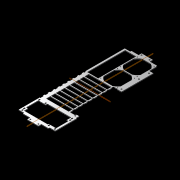
# Autodesk Inventor part: backpanel
Saved by Autodesk Inventor 2018 (Build 220112000, 112)
## iProperties
Created: 2019-10-14
Part Number: backpanel
Material: アルミニウム 6061
Document SubType Name: Modeling
Designer: gisen
Density: 2.7 g/cm^3
Appearance: アルミニウム - フラット
Author: gisen
Autodesk Inventor part; units mm, degrees
ref_plane "XY Plane" through (0, 0, 0) normal (0, 0, 1) x (1, 0, 0)
sketch "スケッチ1" plane through (0, 0, 0) normal (0, 0, 1) x (1, 0, 0)
  line L0 (-55, -225) -> (55, -225) construction
  line L1 (55, -225) -> (55, 225) construction
  line L2 (55, 225) -> (-55, 225) construction
  line L3 (-55, 225) -> (-55, -225) construction
  line L4 (-55, -225) -> (55, 225) construction
  line L5 (55, -225) -> (-55, 225) construction
  line L6 (-75, 225) -> (-55, 225)
  line L7 (-55, 225) -> (-55, 242.5)
  line L8 (-55, 242.5) -> (55, 242.5)
  line L9 (55, 242.5) -> (55, 225)
  line L10 (55, 225) -> (75, 225)
  line L11 (75, 225) -> (75, -225)
  line L12 (75, -225) -> (55, -225)
  line L13 (55, -225) -> (55, -242.5)
  line L14 (55, -242.5) -> (-55, -242.5)
  line L15 (-55, -242.5) -> (-55, -225)
  line L16 (-55, -225) -> (-75, -225)
  line L17 (-75, -225) -> (-75, 225)
  line L18 (-65, 235) -> (65, 235) construction
  line L19 (65, 235) -> (65, -235) construction
  line L20 (65, -235) -> (-65, -235) construction
  line L21 (-65, -235) -> (-65, 235) construction
  circle A0 centre (-45, 235) radius 2.25
  circle A1 centre (-65, 215) radius 2.25
  line L22 (0, 0) -> (0, 242.5) construction
  line L23 (0, 0) -> (-75, 0) construction
  circle A2 centre (45, 235) radius 2.25
  circle A3 centre (65, 215) radius 2.25
  circle A4 centre (-45, -235) radius 2.25
  circle A5 centre (-65, -215) radius 2.25
  circle A6 centre (45, -235) radius 2.25
  circle A7 centre (65, -215) radius 2.25
  dimension "d0" = 110
  dimension "d1" = 450
  dimension "d2" = 17.5
  dimension "d3" = 17.5
  dimension "d4" = 20
  dimension "d5" = 20
  dimension "d6" = 10
  dimension "d7" = 10
  dimension "d8" = 10
  dimension "d9" = 10
  dimension "d10" = 4.5
  dimension "d11" = 10
  dimension "d12" = 10
  constraints: 48 end point, 8 centre point, 6 perpendicular, 6 point on line, 6 symmetric about line, 5 parallel, 4 midpoint, 4 vertical, 3 horizontal, 1 equal radius, 6 other
  measures "d0" distance of L2.end L1.end
  measures "d1" distance of L1.end L0.end
  measures "d2" distance of L8.end L1.end
  measures "d3" distance of L0.end L13.end
  measures "d4" distance of L1.end L10.end
  measures "d5" distance of L6.start L2.end
  measures "d6" distance between parallel lines of L2 L18
  measures "d7" distance between parallel lines of L3 L21
  measures "d8" distance between parallel lines of L0 L20
  measures "d9" distance between parallel lines of L1 L19
  measures "d10" diameter of A0
  measures "d11" distance from line of L7 A0.centre
  measures "d12" distance from line of A1.centre L6
extrude "押し出し1" add sketch "スケッチ1" along normal blind 3 contours L6 L7 L8 L9 L10 L11 L12 L13 L14 L15 L16 L17 | A1 | A5 | A7
sketch "スケッチ2" plane through (0, 0, 3) normal (0, 0, 1) x (1, 0, 0)
  line L0 (-68.059, 218.004) -> (-25.879, 218.004) construction
  line L1 (-69.259, 60.324) -> (-69.259, 216.804) construction
  line L2 (-25.879, 59.124) -> (-68.059, 59.124) construction
  line L3 (-24.679, 216.804) -> (-24.679, 60.324) construction
  line L4 (-24.679, 59.124) -> (-69.259, 59.124) construction
  line L5 (-69.259, 59.124) -> (-69.259, 218.004) construction
  line L6 (-69.259, 218.004) -> (-24.679, 218.004) construction
  line L7 (-24.679, 218.004) -> (-24.679, 59.124) construction
  line L8 (-24.679, 59.124) -> (-69.259, 218.004) construction
  line L9 (-69.259, 59.124) -> (-24.679, 218.004) construction
  line L10 (-69.319, 59.064) -> (-24.619, 59.064)
  line L11 (-24.619, 59.064) -> (-24.619, 218.064)
  line L12 (-24.619, 218.064) -> (-69.319, 218.064)
  line L13 (-69.319, 218.064) -> (-69.319, 59.064)
  line L14 (-69.319, 59.064) -> (-24.619, 218.064) construction
  line L15 (-24.619, 59.064) -> (-69.319, 218.064) construction
  point P0 (0, 0)
  point P1 (-46.969, 138.564)
  point P2 (-46.969, 218.004)
  point P3 (-69.259, 138.564)
  dimension "d16" = 44.7
  dimension "d17" = 159
  constraints: 24 end point, 8 midpoint, 4 parallel, 2 horizontal, 2 perpendicular
  measures "d16" distance of L12.end L11.end
  measures "d17" distance of L11.end L10.end
extrude "押し出し2" cut sketch "スケッチ2" against normal blind 3
sketch "スケッチ3" plane through (0, 0, 3) normal (0, 0, 1) x (1, 0, 0)
  line L0 (-70.088, -102.7387) -> (-77.3126, -102.7387) construction
  line L1 (-77.3126, -92.4517) -> (-70.088, -92.4517) construction
  line L2 (-70.088, -82.3933) -> (-77.3126, -82.3933) construction
  line L3 (-77.3126, -72.1063) -> (-70.088, -72.1063) construction
  line L4 (-70.088, -61.7387) -> (-77.3126, -61.7387) construction
  line L5 (-77.3126, -51.4517) -> (-70.088, -51.4517) construction
  line L6 (-70.088, -41.3933) -> (-77.3126, -41.3933) construction
  line L7 (-77.3126, -31.1063) -> (-70.088, -31.1063) construction
  line L8 (-70.088, -20.7387) -> (-77.3126, -20.7387) construction
  line L9 (-77.3126, -10.4517) -> (-70.088, -10.4517) construction
  line L10 (-70.088, -0.3933) -> (-77.3126, -0.3933) construction
  line L11 (-77.3126, 9.8937) -> (-70.088, 9.8937) construction
  line L12 (-70.088, 20.2613) -> (-77.3126, 20.2613) construction
  line L13 (-77.3126, 30.5483) -> (-70.088, 30.5483) construction
  line L14 (-70.088, 40.6067) -> (-77.3126, 40.6067) construction
  line L15 (-77.3126, 50.8937) -> (-70.088, 50.8937) construction
  line L16 (-75, 225) -> (-75, -225) construction
  line L17 (-75, 56.064) -> (-78, 56.064)
  line L18 (-78, 56.064) -> (-78, 225)
  line L19 (-78, 225) -> (-75, 225)
  line L20 (-75, 225) -> (-75, 56.064)
  line L21 (-24.619, 59.064) -> (-69.319, 59.064) projected
  line L22 (-75, -102.7387) -> (-78, -102.7387)
  line L23 (-78, -102.7387) -> (-78, -92.4517)
  line L24 (-78, -92.4517) -> (-75, -92.4517)
  line L25 (-75, -92.4517) -> (-75, -102.7387)
  line L26 (-75, -82.3933) -> (-78, -82.3933)
  line L27 (-78, -82.3933) -> (-78, -72.1063)
  line L28 (-78, -72.1063) -> (-75, -72.1063)
  line L29 (-75, -72.1063) -> (-75, -82.3933)
  line L30 (-75, -61.7387) -> (-78, -61.7387)
  line L31 (-78, -61.7387) -> (-78, -51.4517)
  line L32 (-78, -51.4517) -> (-75, -51.4517)
  line L33 (-75, -51.4517) -> (-75, -61.7387)
  line L34 (-75, -41.3933) -> (-78, -41.3933)
  line L35 (-78, -41.3933) -> (-78, -31.1063)
  line L36 (-78, -31.1063) -> (-75, -31.1063)
  line L37 (-75, -31.1063) -> (-75, -41.3933)
  line L38 (-75, -20.7387) -> (-78, -20.7387)
  line L39 (-78, -20.7387) -> (-78, -10.4517)
  line L40 (-78, -10.4517) -> (-75, -10.4517)
  line L41 (-75, -10.4517) -> (-75, -20.7387)
  line L42 (-75, -0.3933) -> (-78, -0.3933)
  line L43 (-78, -0.3933) -> (-78, 9.8937)
  line L44 (-78, 9.8937) -> (-75, 9.8937)
  line L45 (-75, 9.8937) -> (-75, -0.3933)
  line L46 (-75, 20.2613) -> (-78, 20.2613)
  line L47 (-78, 20.2613) -> (-78, 30.5483)
  line L48 (-78, 30.5483) -> (-75, 30.5483)
  line L49 (-75, 30.5483) -> (-75, 20.2613)
  line L50 (-75, 40.6067) -> (-78, 40.6067)
  line L51 (-78, 40.6067) -> (-78, 50.8937)
  line L52 (-78, 50.8937) -> (-75, 50.8937)
  line L53 (-75, 50.8937) -> (-75, 40.6067)
  line L54 (-78, -112.7971) -> (-75, -112.7971)
  line L55 (-75, -112.7971) -> (-75, -123.0841)
  line L56 (-75, -123.0841) -> (-78, -123.0841)
  line L57 (-78, -123.0841) -> (-78, -112.7971)
  dimension "d20" = 3
  dimension "d21" = 3
  dimension "d184" = 10.287
  dimension "d185" = 10.0584
  dimension "d192" = 10.0584
  constraints: 80 end point, 20 parallel, 16 point on line, 10 equal length, 10 horizontal, 10 perpendicular, 1 vertical alignment, 10 other
  measures "d20" distance of L19.end L18.end
  measures "d21" distance between parallel lines of L21 L17
  measures "d184" distance of L22.end L23.end
  measures "d185" distance between parallel lines of L1 L2
  measures "d192" distance of L54.start L22.end
extrude "押し出し3" add sketch "スケッチ3" against normal blind 3
sketch "スケッチ4" plane through (0, 0, 3) normal (0, 0, 1) x (1, 0, 0)
  line L0 (-67, 211.554) -> (-67, -85.626) construction
  line L1 (-78, 50.8937) -> (-78, 40.6067) construction
  line L2 (-78, 30.5483) -> (-78, 20.2613) construction
  line L3 (-78, 9.8937) -> (-78, -0.3933) construction
  line L4 (-78, -10.4517) -> (-78, -20.7387) construction
  line L5 (-78, -31.1063) -> (-78, -41.3933) construction
  line L6 (-78, -51.4517) -> (-78, -61.7387) construction
  line L7 (-78, -72.1063) -> (-78, -82.3933) construction
  line L8 (-78, -92.4517) -> (-78, -102.7387) construction
  line L9 (-78, 45.7502) -> (-12.1, 45.7502) construction
  line L10 (-58.94, 37.8102) -> (34.74, 37.8102)
  line L11 (34.74, 37.8102) -> (34.74, 53.6902) construction
  line L12 (34.74, 53.6902) -> (-58.94, 53.6902)
  line L13 (-58.94, 53.6902) -> (-58.94, 37.8102)
  line L14 (-58.94, 37.8102) -> (34.74, 53.6902) construction
  line L15 (34.74, 37.8102) -> (-58.94, 53.6902) construction
  line L16 (34.74, 53.6902) -> (34.74, 50.5152)
  line L17 (34.74, 50.5152) -> (35.02, 50.5152)
  line L18 (35.02, 50.5152) -> (35.02, 40.9852)
  line L19 (35.02, 40.9852) -> (34.74, 40.9852)
  line L20 (34.74, 40.9852) -> (34.74, 37.8102)
  line L21 (42.72, 50.3792) -> (42.72, 57.7992) construction
  line L22 (-75, 30.5483) -> (-78, 30.5483) construction
  line L23 (-75, 50.8937) -> (-78, 50.8937) construction
  line L24 (-58.94, 17.4648) -> (34.74, 17.4648)
  line L25 (-58.94, 33.3448) -> (-58.94, 17.4648)
  line L26 (34.74, 33.3448) -> (-58.94, 33.3448)
  line L27 (34.74, 33.3448) -> (34.74, 30.1698)
  line L28 (34.74, 30.1698) -> (35.02, 30.1698)
  line L29 (35.02, 30.1698) -> (35.02, 20.6398)
  line L30 (35.02, 20.6398) -> (34.74, 20.6398)
  line L31 (34.74, 20.6398) -> (34.74, 17.4648)
  line L32 (-58.94, -2.8806) -> (34.74, -2.8806)
  line L33 (-58.94, 12.9994) -> (-58.94, -2.8806)
  line L34 (34.74, 12.9994) -> (-58.94, 12.9994)
  line L35 (34.74, 12.9994) -> (34.74, 9.8244)
  line L36 (34.74, 9.8244) -> (35.02, 9.8244)
  line L37 (35.02, 9.8244) -> (35.02, 0.2944)
  line L38 (35.02, 0.2944) -> (34.74, 0.2944)
  line L39 (34.74, 0.2944) -> (34.74, -2.8806)
  line L40 (-58.94, -23.226) -> (34.74, -23.226)
  line L41 (-58.94, -7.346) -> (-58.94, -23.226)
  line L42 (34.74, -7.346) -> (-58.94, -7.346)
  line L43 (34.74, -7.346) -> (34.74, -10.521)
  line L44 (34.74, -10.521) -> (35.02, -10.521)
  line L45 (35.02, -10.521) -> (35.02, -20.051)
  line L46 (35.02, -20.051) -> (34.74, -20.051)
  line L47 (34.74, -20.051) -> (34.74, -23.226)
  line L48 (-58.94, -43.5714) -> (34.74, -43.5714)
  line L49 (-58.94, -27.6914) -> (-58.94, -43.5714)
  line L50 (34.74, -27.6914) -> (-58.94, -27.6914)
  line L51 (34.74, -27.6914) -> (34.74, -30.8664)
  line L52 (34.74, -30.8664) -> (35.02, -30.8664)
  line L53 (35.02, -30.8664) -> (35.02, -40.3964)
  line L54 (35.02, -40.3964) -> (34.74, -40.3964)
  line L55 (34.74, -40.3964) -> (34.74, -43.5714)
  line L56 (-58.94, -63.9168) -> (34.74, -63.9168)
  line L57 (-58.94, -48.0368) -> (-58.94, -63.9168)
  line L58 (34.74, -48.0368) -> (-58.94, -48.0368)
  line L59 (34.74, -48.0368) -> (34.74, -51.2118)
  line L60 (34.74, -51.2118) -> (35.02, -51.2118)
  line L61 (35.02, -51.2118) -> (35.02, -60.7418)
  line L62 (35.02, -60.7418) -> (34.74, -60.7418)
  line L63 (34.74, -60.7418) -> (34.74, -63.9168)
  line L64 (-58.94, -84.2622) -> (34.74, -84.2622)
  line L65 (-58.94, -68.3822) -> (-58.94, -84.2622)
  line L66 (34.74, -68.3822) -> (-58.94, -68.3822)
  line L67 (34.74, -68.3822) -> (34.74, -71.5572)
  line L68 (34.74, -71.5572) -> (35.02, -71.5572)
  line L69 (35.02, -71.5572) -> (35.02, -81.0872)
  line L70 (35.02, -81.0872) -> (34.74, -81.0872)
  line L71 (34.74, -81.0872) -> (34.74, -84.2622)
  line L72 (-58.94, -104.6076) -> (34.74, -104.6076)
  line L73 (-58.94, -88.7276) -> (-58.94, -104.6076)
  line L74 (34.74, -88.7276) -> (-58.94, -88.7276)
  line L75 (34.74, -88.7276) -> (34.74, -91.9026)
  line L76 (34.74, -91.9026) -> (35.02, -91.9026)
  line L77 (35.02, -91.9026) -> (35.02, -101.4326)
  line L78 (35.02, -101.4326) -> (34.74, -101.4326)
  line L79 (34.74, -101.4326) -> (34.74, -104.6076)
  line L80 (75, -225) -> (75, 225) projected
  line L81 (42.22, -124.469) -> (75, -124.469)
  line L82 (75, -124.469) -> (75, 58.3992)
  line L83 (75, 58.3992) -> (42.22, 58.3992)
  line L84 (42.22, 58.3992) -> (42.22, -124.469)
  line L85 (42.82, 57.8992) -> (43.62, 57.8992) projected
  line L86 (-58.94, -124.953) -> (34.74, -124.953)
  line L87 (-58.94, -109.073) -> (-58.94, -124.953)
  line L88 (34.74, -109.073) -> (-58.94, -109.073)
  line L89 (34.74, -109.073) -> (34.74, -112.248)
  line L90 (34.74, -112.248) -> (35.02, -112.248)
  line L91 (35.02, -112.248) -> (35.02, -121.778)
  line L92 (35.02, -121.778) -> (34.74, -121.778)
  line L93 (34.74, -121.778) -> (34.74, -124.953)
  point P0 (35.02, 45.7502)
  point P1 (35.02, 25.4048)
  point P2 (35.02, 5.0594)
  point P3 (35.02, -15.286)
  point P4 (35.02, -35.6314)
  point P5 (35.02, -55.9768)
  point P6 (35.02, -76.3222)
  point P7 (35.02, -96.6676)
  point P8 (35.02, -117.013)
  dimension "d24" = 8.06
  dimension "d25" = 93.68
  dimension "d26" = 15.88
  dimension "d27" = 9.53
  dimension "d28" = 7.7
  dimension "d29" = 20.3454
  dimension "d32" = 20.3454
  dimension "d38" = 0.5
  dimension "d97" = 0.5
  dimension "d188" = 0.484
  constraints: 160 end point, 4 horizontal, 4 midpoint, 4 parallel, 4 perpendicular, 4 point on line, 1 collinear, 1 vertical, 136 other
  measures "d24" distance between parallel lines of L0 L13
  measures "d25" distance of L11.end L12.end
  measures "d26" distance of L12.end L10.start
  measures "d27" distance of L17.end L18.end
  measures "d28" distance between parallel lines of L18 L21
  measures "d29" distance between parallel lines of L22 L23
  measures "d32" distance of L10.start L24.start
  measures "d38" distance from line of L21 L83.end
  measures "d97" distance between parallel lines of L85 L83
  measures "d188" distance between parallel lines of L86 L81
extrude "押し出し4" cut sketch "スケッチ4" against normal blind 3
sketch "スケッチ5" plane through (0, 0, 3) normal (0, 0, 1) x (1, 0, 0)
  line L0 (75, -132.8) -> (75, -206.1029) construction
  line L1 (-73.8, -131.6) -> (73.8, -131.6) construction
  line L2 (-75, -137.8) -> (-75, -211.1029) construction
  line L3 (73, -217) -> (-73, -217) construction
  line L4 (0, -131.6) -> (0, -217) construction
  line L5 (-70, -137.4) -> (-70, -140.4) construction
  line L6 (-71.75, -137.4) -> (-71.75, -140.4)
  line L7 (-68.25, -140.4) -> (-68.25, -137.4)
  arc A0 (-68.25, -137.4) -> (-71.75, -137.4) centre (-70, -137.4) ccw
  arc A1 (-71.75, -140.4) -> (-68.25, -140.4) centre (-70, -140.4) ccw
  line L8 (-44, -137.2) -> (-44, -140.2) construction
  line L9 (-45.75, -137.2) -> (-45.75, -140.2)
  line L10 (-42.25, -140.2) -> (-42.25, -137.2)
  arc A2 (-42.25, -137.2) -> (-45.75, -137.2) centre (-44, -137.2) ccw
  arc A3 (-45.75, -140.2) -> (-42.25, -140.2) centre (-44, -140.2) ccw
  line L11 (-70, -201.4) -> (-70, -204.4) construction
  line L12 (-72, -201.4) -> (-72, -204.4)
  line L13 (-68, -204.4) -> (-68, -201.4)
  arc A4 (-68, -201.4) -> (-72, -201.4) centre (-70, -201.4) ccw
  arc A5 (-72, -204.4) -> (-68, -204.4) centre (-70, -204.4) ccw
  line L14 (-68, -211.2) -> (-68, -214.2) construction
  line L15 (-69.75, -211.2) -> (-69.75, -214.2)
  line L16 (-66.25, -214.2) -> (-66.25, -211.2)
  arc A6 (-66.25, -211.2) -> (-69.75, -211.2) centre (-68, -211.2) ccw
  arc A7 (-69.75, -214.2) -> (-66.25, -214.2) centre (-68, -214.2) ccw
  line L17 (68, -137.4) -> (68, -140.4) construction
  line L18 (66.25, -137.4) -> (66.25, -140.4)
  line L19 (69.75, -140.4) -> (69.75, -137.4)
  arc A8 (69.75, -137.4) -> (66.25, -137.4) centre (68, -137.4) ccw
  arc A9 (66.25, -140.4) -> (69.75, -140.4) centre (68, -140.4) ccw
  line L20 (70, -147.2) -> (70, -150.2) construction
  line L21 (68.25, -147.2) -> (68.25, -150.2)
  line L22 (71.75, -150.2) -> (71.75, -147.2)
  arc A10 (71.75, -147.2) -> (68.25, -147.2) centre (70, -147.2) ccw
  arc A11 (68.25, -150.2) -> (71.75, -150.2) centre (70, -150.2) ccw
  line L23 (70, -211.2) -> (70, -214.2) construction
  line L24 (68.25, -211.2) -> (68.25, -214.2)
  line L25 (71.75, -214.2) -> (71.75, -211.2)
  arc A12 (71.75, -211.2) -> (68.25, -211.2) centre (70, -211.2) ccw
  arc A13 (68.25, -214.2) -> (71.75, -214.2) centre (70, -214.2) ccw
  line L26 (44, -211.4) -> (44, -214.4) construction
  line L27 (42.25, -211.4) -> (42.25, -214.4)
  line L28 (45.75, -214.4) -> (45.75, -211.4)
  arc A14 (45.75, -211.4) -> (42.25, -211.4) centre (44, -211.4) ccw
  arc A15 (42.25, -214.4) -> (45.75, -214.4) centre (44, -214.4) ccw
  line L29 (-69, -144.4) -> (-37.5, -144.4)
  line L30 (-37.5, -144.4) -> (-37.5, -137.6)
  line L31 (-37.5, -137.6) -> (61.5, -137.6)
  line L32 (61.5, -137.6) -> (61.5, -156.7)
  line L33 (61.5, -156.7) -> (69, -156.7)
  line L34 (69, -156.7) -> (69, -207.4)
  line L35 (69, -207.4) -> (37.5, -207.4)
  line L36 (37.5, -207.4) -> (37.5, -211)
  line L37 (37.5, -211) -> (-61.5, -211)
  line L38 (-61.5, -211) -> (-61.5, -194.9)
  line L39 (-61.5, -194.9) -> (-69, -194.9)
  line L40 (-69, -194.9) -> (-69, -144.4)
  point P0 (0, 0)
  point P1 (0, -174.3)
  point P2 (-70, -202.9)
  point P3 (-68, -212.7)
  point P4 (68, -138.9)
  point P5 (70, -148.7)
  point P6 (70, -212.7)
  point P7 (44, -212.9)
  dimension "d44" = 180
  dimension "d46" = 3.5
  dimension "d47" = 3
  dimension "d48" = 6
  dimension "d49" = 6
  dimension "d50" = 4
  dimension "d51" = 6.5
  dimension "d52" = 6.5
  dimension "d53" = 6.5
  dimension "d54" = 6
  dimension "d55" = 4
  dimension "d56" = 6.5
  dimension "d57" = 6
  dimension "d58" = 6.5
  dimension "d59" = 6.5
  dimension "d195" = 36.7
  dimension "d196" = 0.2
  dimension "d197" = 5.8
  dimension "d198" = 7
  dimension "d199" = 3.6
  dimension "d200" = 19.1
  dimension "d201" = 1
  dimension "d202" = 1
  dimension "d203" = 31.5
  constraints: 92 end point, 32 point on circle, 32 tangent, 16 centre point, 12 perpendicular, 11 parallel, 9 midpoint, 7 equal length, 6 equal radius, 4 vertical, 1 horizontal, 1 point on line, 5 other
  measures "d46" diameter of A1
  measures "d47" distance of L7.start L7.end
  measures "d48" distance between parallel lines of L2 L40
  measures "d49" distance between parallel lines of L0 L34
  measures "d50" distance from line of L29 L5.end
  measures "d51" distance from line of L8.end L30
  measures "d52" distance from line of L17.end L32
  measures "d53" distance from line of L33 L20.end
  measures "d54" distance between parallel lines of L31 L1
  measures "d55" distance from line of L26.start L35
  measures "d56" distance from line of L26.start L36
  measures "d57" distance between parallel lines of L3 L37
  measures "d58" distance from line of L14.start L38
  measures "d59" distance from line of L39 L11.start
  measures "d195" distance from line of point (0, -174.3) L31
  measures "d196" distance from line of L31 L5.start
  measures "d197" distance from line of L17.start L1
  measures "d198" distance between parallel lines of L17 L0
  measures "d199" distance of L35.end L36.end
  measures "d200" distance of L31.end L32.end
  measures "d201" distance from line of L20.end L34
  measures "d202" distance from line of L5.end L40
  measures "d203" distance of L29.start L29.end
extrude "押し出し5" cut sketch "スケッチ5" against normal blind 3
sketch "スケッチ6" plane through (0, 0, 3) normal (0, 0, 1) x (1, 0, 0)
  line L0 (-75, -225) -> (-55, -225) projected
  line L1 (-75, -225) -> (-78, -225)
  line L2 (-78, -225) -> (-78, -129.6)
  line L3 (-78, -129.6) -> (-75, -129.6)
  line L4 (-75, -129.6) -> (-75, -225)
  line L5 (-78, -102.7387) -> (-75, -102.7387) projected
  line L6 (-37.5, -137.6) -> (61.5, -137.6) projected
  point P0 (0, 0)
  point P1 (-36.2992, -140.6)
  point P2 (58.5, -140.6)
  point P3 (-24.619, -122.5995)
  point P4 (-58.94, -225)
  point P5 (-75, -337.7387)
  point P6 (42.22, -122.5995)
  point P7 (61.5, -137.6)
  point P8 (-24.619, -140.6)
  dimension "d63" = 8
  constraints: 8 end point, 2 horizontal, 2 parallel, 1 perpendicular, 2 other
extrude "押し出し6" add sketch "スケッチ6" against normal blind 3
sketch "スケッチ7" plane through (0, 0, 3) normal (0, 0, 1) x (1, 0, 0)
  line L0 (56.381, 140.3992) -> (-23.619, 140.3992) construction
  line L1 (-23.619, 140.3992) -> (-23.619, 60.3992) construction
  line L2 (-23.619, 60.3992) -> (56.381, 60.3992) construction
  line L3 (56.381, 60.3992) -> (56.381, 140.3992) construction
  line L4 (56.381, 140.3992) -> (-23.619, 60.3992) construction
  line L5 (-23.619, 140.3992) -> (56.381, 60.3992) construction
  line L6 (-23.619, 223.3992) -> (56.381, 223.3992) construction
  line L7 (56.381, 223.3992) -> (56.381, 143.3992) construction
  line L8 (56.381, 143.3992) -> (-23.619, 143.3992) construction
  line L9 (-23.619, 143.3992) -> (-23.619, 223.3992) construction
  line L10 (-23.619, 223.3992) -> (56.381, 143.3992) construction
  line L11 (56.381, 223.3992) -> (-23.619, 143.3992) construction
  line L12 (42.22, 58.3992) -> (75, 58.3992) construction
  line L13 (-24.619, 218.064) -> (-24.619, 59.064) construction
  circle A0 centre (16.381, 100.3992) radius 42.5 construction
  line L14 (-22.419, 61.5992) -> (55.181, 61.5992) construction
  line L15 (55.181, 61.5992) -> (55.181, 139.1992) construction
  line L16 (55.181, 139.1992) -> (-22.419, 139.1992) construction
  line L17 (-22.419, 139.1992) -> (-22.419, 61.5992) construction
  line L18 (-22.419, 61.5992) -> (55.181, 139.1992) construction
  line L19 (55.181, 61.5992) -> (-22.419, 139.1992) construction
  line L20 (-19.369, 64.6492) -> (52.131, 64.6492) construction
  line L21 (52.131, 64.6492) -> (52.131, 136.1492) construction
  line L22 (52.131, 136.1492) -> (-19.369, 136.1492) construction
  line L23 (-19.369, 136.1492) -> (-19.369, 64.6492) construction
  line L24 (-19.369, 64.6492) -> (52.131, 136.1492) construction
  line L25 (52.131, 64.6492) -> (-19.369, 136.1492) construction
  arc A1 (-0.9629, 139.1992) -> (-22.419, 117.7431) centre (16.381, 100.3992) ccw
  arc A2 (55.181, 117.7431) -> (33.7249, 139.1992) centre (16.381, 100.3992) ccw
  arc A3 (-22.419, 83.0554) -> (-0.9629, 61.5992) centre (16.381, 100.3992) ccw
  arc A4 (33.7249, 61.5992) -> (55.181, 83.0554) centre (16.381, 100.3992) ccw
  line L26 (-22.419, 117.7431) -> (-22.419, 83.0554)
  line L27 (-0.9629, 61.5992) -> (33.7249, 61.5992)
  line L28 (55.181, 117.7431) -> (55.181, 83.0554)
  line L29 (-0.9629, 139.1992) -> (33.7249, 139.1992)
  circle A5 centre (-19.369, 136.1492) radius 1.2
  circle A6 centre (52.131, 136.1492) radius 1.2
  circle A7 centre (-19.369, 64.6492) radius 1.2
  circle A8 centre (52.131, 64.6492) radius 1.2
  circle A9 centre (-19.369, 219.1492) radius 1.2
  arc A10 (-0.9629, 222.1992) -> (-22.419, 200.7431) centre (16.381, 183.3992) ccw
  line L30 (-0.9629, 222.1992) -> (33.7249, 222.1992)
  arc A11 (55.181, 200.7431) -> (33.7249, 222.1992) centre (16.381, 183.3992) ccw
  circle A12 centre (52.131, 219.1492) radius 1.2
  line L31 (55.181, 200.7431) -> (55.181, 166.0554)
  arc A13 (33.7249, 144.5992) -> (55.181, 166.0554) centre (16.381, 183.3992) ccw
  line L32 (-0.9629, 144.5992) -> (33.7249, 144.5992)
  circle A14 centre (52.131, 147.6492) radius 1.2
  circle A15 centre (-19.369, 147.6492) radius 1.2
  arc A16 (-22.419, 166.0554) -> (-0.9629, 144.5992) centre (16.381, 183.3992) ccw
  line L33 (-22.419, 200.7431) -> (-22.419, 166.0554)
  point P0 (0, 0)
  point P1 (16.381, 183.3992)
  point P2 (-24.619, -104.6076)
  point P3 (-24.619, -122.5995)
  point P4 (69.0004, -176.6008)
  point P5 (-24.619, -23.226)
  point P6 (-24.619, -27.6914)
  dimension "d74" = 85
  dimension "d66" = 80
  dimension "d67" = 80
  dimension "d68" = 80
  dimension "d69" = 80
  dimension "d70" = 3
  dimension "d71" = 2
  dimension "d73" = 1
  dimension "d78" = 71.5
  dimension "d79" = 71.5
  dimension "d80" = 2.4
  dimension "d81" = 77.6
  dimension "d84" = 83
  constraints: 64 end point, 16 centre point, 16 point on circle, 12 midpoint, 10 coincident, 9 parallel, 9 point on line, 6 perpendicular, 4 horizontal, 3 equal radius, 1 collinear, 1 vertical, 39 other
  measures "d66" distance of L2.end L1.end
  measures "d67" distance of L1.end L0.end
  measures "d68" distance of L7.end L8.end
  measures "d69" distance of L6.end L7.end
  measures "d70" distance between parallel lines of L0 L8
  measures "d73" distance between parallel lines of L13 L9
  measures "d78" distance of L22.end L21.end
  measures "d79" distance of L21.end L20.end
  measures "d80" diameter of A5
  measures "d81" distance of L15.end L16.end
  measures "d84" distance of A5.centre A9.centre
extrude "押し出し7" cut sketch "スケッチ7" against normal blind 3
sketch "スケッチ8" plane through (0, 0, 3) normal (0, 0, 1) x (1, 0, 0)
  line L0 (-19.619, 122.988) -> (-22.419, 122.988)
  line L1 (-22.419, 122.988) -> (-22.419, 77.8105)
  line L2 (-22.419, 77.8105) -> (-19.619, 77.8105)
  line L3 (-19.619, 77.8105) -> (-19.619, 122.988)
  line L4 (-22.419, 83.0554) -> (-22.419, 117.7431) projected
  line L5 (-19.619, 160.8105) -> (-22.419, 160.8105)
  line L6 (-22.419, 160.8105) -> (-22.419, 205.988)
  line L7 (-22.419, 205.988) -> (-19.619, 205.988)
  line L8 (-19.619, 205.988) -> (-19.619, 160.8105)
  line L9 (-22.419, 166.0554) -> (-22.419, 200.7431) projected
  line L10 (16.381, 183.3992) -> (16.381, 100.3992) construction
  line L11 (52.381, 122.988) -> (55.181, 122.988)
  line L12 (55.181, 122.988) -> (55.181, 77.8105)
  line L13 (55.181, 77.8105) -> (52.381, 77.8105)
  line L14 (52.381, 77.8105) -> (52.381, 122.988)
  line L15 (55.181, 83.0554) -> (55.181, 117.7431)
  line L16 (52.381, 160.8105) -> (55.181, 160.8105)
  line L17 (55.181, 160.8105) -> (55.181, 205.988)
  line L18 (55.181, 205.988) -> (52.381, 205.988)
  line L19 (52.381, 205.988) -> (52.381, 160.8105)
  line L20 (55.181, 166.0554) -> (55.181, 200.7431)
  arc A0 (-0.9629, 222.1992) -> (-22.419, 200.7431) centre (16.381, 183.3992) ccw construction
  arc A1 (-22.419, 166.0554) -> (-0.9629, 144.5992) centre (16.381, 183.3992) ccw construction
  arc A2 (-0.9629, 139.1992) -> (-22.419, 117.7431) centre (16.381, 100.3992) ccw construction
  arc A3 (-22.419, 83.0554) -> (-0.9629, 61.5992) centre (16.381, 100.3992) ccw construction
  dimension "d92" = 2.8
  constraints: 38 end point, 12 symmetric about line, 6 point on line, 5 parallel, 4 point on circle, 2 coincident, 2 horizontal, 2 perpendicular
  measures "d92" distance between parallel lines of L1 L3
extrude "押し出し8" add sketch "スケッチ8" against normal blind 3
sketch "スケッチ9" plane through (0, 0, 3) normal (0, 0, 1) x (1, 0, 0)
  line L0 (42.82, -5.4782) -> (42.82, -6.9799) construction
  line L1 (43.62, 34.771) -> (39.12, 34.771) construction
  line L2 (39.12, 34.771) -> (39.12, -6.229) construction
  line L3 (39.12, 55.271) -> (40.67, 55.271) construction
  line L4 (39.12, 52.271) -> (42.22, 52.271)
  line L5 (42.22, 52.271) -> (42.22, 58.271)
  line L6 (42.22, 58.271) -> (39.12, 58.271)
  line L7 (39.12, 58.271) -> (39.12, 52.271)
  line L8 (39.12, 52.271) -> (42.22, 58.271) construction
  line L9 (42.22, 52.271) -> (39.12, 58.271) construction
  line L10 (42.22, 31.771) -> (39.12, 31.771)
  line L11 (39.12, 31.771) -> (39.12, 37.771)
  line L12 (39.12, 37.771) -> (42.22, 37.771)
  line L13 (42.22, 37.771) -> (42.22, 31.771)
  line L14 (42.22, 31.771) -> (39.12, 37.771) construction
  line L15 (39.12, 31.771) -> (42.22, 37.771) construction
  line L16 (42.22, 17.271) -> (39.12, 17.271)
  line L17 (39.12, 14.271) -> (40.67, 14.271) construction
  line L18 (42.22, 11.271) -> (42.22, 17.271)
  line L19 (39.12, 17.271) -> (39.12, 11.271)
  line L20 (39.12, 11.271) -> (42.22, 17.271) construction
  line L21 (39.12, 11.271) -> (42.22, 11.271)
  line L22 (42.22, 11.271) -> (39.12, 17.271) construction
  line L23 (42.22, -9.229) -> (39.12, -9.229)
  line L24 (42.22, -3.229) -> (42.22, -9.229)
  line L25 (39.12, -9.229) -> (39.12, -3.229)
  line L26 (42.22, -9.229) -> (39.12, -3.229) construction
  line L27 (39.12, -9.229) -> (42.22, -3.229) construction
  line L28 (39.12, -3.229) -> (42.22, -3.229)
  line L29 (43.62, -6.229) -> (39.12, -6.229) construction
  line L30 (42.22, -23.729) -> (39.12, -23.729)
  line L31 (39.12, -26.729) -> (40.67, -26.729) construction
  line L32 (42.22, -29.729) -> (42.22, -23.729)
  line L33 (39.12, -23.729) -> (39.12, -29.729)
  line L34 (39.12, -29.729) -> (42.22, -23.729) construction
  line L35 (39.12, -29.729) -> (42.22, -29.729)
  line L36 (42.22, -29.729) -> (39.12, -23.729) construction
  line L37 (42.22, -50.229) -> (39.12, -50.229)
  line L38 (42.22, -44.229) -> (42.22, -50.229)
  line L39 (39.12, -50.229) -> (39.12, -44.229)
  line L40 (42.22, -50.229) -> (39.12, -44.229) construction
  line L41 (39.12, -50.229) -> (42.22, -44.229) construction
  line L42 (39.12, -44.229) -> (42.22, -44.229)
  line L43 (43.62, -47.229) -> (39.12, -47.229) construction
  line L44 (42.22, -64.729) -> (39.12, -64.729)
  line L45 (39.12, -67.729) -> (40.67, -67.729) construction
  line L46 (42.22, -70.729) -> (42.22, -64.729)
  line L47 (39.12, -64.729) -> (39.12, -70.729)
  line L48 (39.12, -70.729) -> (42.22, -64.729) construction
  line L49 (39.12, -70.729) -> (42.22, -70.729)
  line L50 (42.22, -70.729) -> (39.12, -64.729) construction
  line L51 (42.22, -91.229) -> (39.12, -91.229)
  line L52 (42.22, -85.229) -> (42.22, -91.229)
  line L53 (39.12, -91.229) -> (39.12, -85.229)
  line L54 (42.22, -91.229) -> (39.12, -85.229) construction
  line L55 (39.12, -91.229) -> (42.22, -85.229) construction
  line L56 (39.12, -85.229) -> (42.22, -85.229)
  line L57 (43.62, -88.229) -> (39.12, -88.229) construction
  line L58 (42.82, -6.9809) -> (42.82, -9.1612) projected
  line L59 (42.82, -3.3193) -> (42.82, -5.4782) projected
  line L60 (42.22, -105.729) -> (39.12, -105.729)
  line L61 (39.12, -108.729) -> (40.67, -108.729) construction
  line L62 (42.22, -111.729) -> (42.22, -105.729)
  line L63 (39.12, -105.729) -> (39.12, -111.729)
  line L64 (39.12, -111.729) -> (42.22, -105.729) construction
  line L65 (39.12, -111.729) -> (42.22, -111.729)
  line L66 (42.22, -111.729) -> (39.12, -105.729) construction
  line L67 (42.22, -132.229) -> (39.12, -132.229)
  line L68 (42.22, -126.229) -> (42.22, -132.229)
  line L69 (39.12, -132.229) -> (39.12, -126.229)
  line L70 (42.22, -132.229) -> (39.12, -126.229) construction
  line L71 (39.12, -132.229) -> (42.22, -126.229) construction
  line L72 (39.12, -126.229) -> (42.22, -126.229)
  line L73 (43.62, -129.229) -> (39.12, -129.229) construction
  point P0 (43.62, 35.5218)
  point P1 (43.62, 34.0201)
  point P2 (43.62, 54.5718)
  point P3 (43.62, 57.7992)
  point P4 (42.22, 58.3992)
  point P5 (40.67, 34.771)
  point P6 (43.6196, 1.4626)
  point P7 (43.62, 13.5718)
  point P8 (43.62, 16.7992)
  point P9 (42.22, 17.3992)
  point P10 (43.62, -6.9799)
  point P11 (40.67, -6.229)
  point P12 (43.6196, -17.0164)
  point P13 (43.62, -5.4782)
  point P14 (43.6196, -13.2695)
  point P15 (43.6196, -19.1967)
  point P16 (43.6196, -39.5374)
  point P17 (43.62, -27.4282)
  point P18 (43.62, -24.2008)
  point P19 (42.22, -23.6008)
  point P20 (43.62, -47.9799)
  point P21 (40.67, -47.229)
  point P22 (43.6196, -58.0164)
  point P23 (43.62, -46.4782)
  point P24 (43.6196, -54.2695)
  point P25 (43.6196, -60.1967)
  point P26 (43.6196, -80.5374)
  point P27 (43.62, -68.4282)
  point P28 (43.62, -65.2008)
  point P29 (42.22, -64.6008)
  point P30 (43.62, -88.9799)
  point P31 (40.67, -88.229)
  point P32 (43.6196, -99.0164)
  point P33 (43.62, -87.4782)
  point P34 (43.6196, -95.2695)
  point P35 (43.6196, -101.1967)
  point P36 (43.6196, -121.5374)
  point P37 (43.62, -109.4282)
  point P38 (43.62, -106.2008)
  point P39 (42.22, -105.6008)
  point P40 (43.62, -129.9799)
  point P41 (40.67, -129.229)
  point P42 (43.6196, -140.0164)
  point P43 (43.62, -128.4782)
  point P44 (43.6196, -136.2695)
  point P45 (43.6196, -142.1967)
  dimension "d105" = 41
  dimension "d101" = 41
  dimension "d102" = 6
  constraints: 142 end point, 20 midpoint, 5 point on line, 4 horizontal, 4 parallel, 2 perpendicular, 1 collinear, 1 vertical, 140 other
  measures "d101" distance from line of L2.end L1
  measures "d102" distance of L6.end L4.start
extrude "押し出し9" cut sketch "スケッチ9" against normal blind 3 contours L7 L6 L5 L4 | L10 L11 L12 L13 | L18 L21 L19 L16 | L23 L25 L28 L24 | L32 L35 L33 L30 | L37 L39 L42 L38 | L46 L49 L47 L44 | L51 L53 L56 L52 | L62 L65 L63 L60
sketch "スケッチ10" plane through (0, 0, 3) normal (0, 0, 1) x (1, 0, 0)
  line L0 (42.22, -124.469) -> (40.72, -124.469)
  line L1 (40.72, -124.469) -> (40.72, 59.771)
  line L2 (40.72, 59.771) -> (42.22, 59.771)
  line L3 (42.22, 59.771) -> (42.22, -124.469)
  line L4 (39.12, 58.271) -> (42.22, 58.271) projected
  line L5 (42.22, -124.469) -> (42.22, 58.3992) construction
  line L6 (42.22, -111.729) -> (39.12, -111.729) construction
  line L7 (75, -124.469) -> (42.22, -124.469) construction
  point P0 (0, 0)
  point P1 (-14.8941, -102.9944)
  point P2 (-14.8941, -98.4595)
  point P3 (42.22, 37.771)
  point P4 (42.22, 40.9852)
  point P5 (42.22, 0.2944)
  point P6 (42.22, 192.5163)
  point P7 (42.22, 9.8244)
  point P8 (42.22, 58.3992)
  dimension "d112" = 1.5
  dimension "d149" = 1.5
  dimension "d189" = 12.74
  constraints: 8 end point, 2 parallel, 1 horizontal, 1 perpendicular, 1 point on line, 2 other
  measures "d112" distance of L0.start L0.end
  measures "d149" distance between parallel lines of L4 L2
  measures "d189" distance between parallel lines of L0 L6
extrude "押し出し10" cut sketch "スケッチ10" against normal blind 3
sketch "スケッチ11" plane through (0, 0, 3) normal (0, 0, 1) x (1, 0, 0)
  circle A0 centre (65, 68.3992) radius 2.25
  circle A1 centre (65, 141.8992) radius 2.25
  line L0 (-55, 230) -> (-24.5, 230)
  line L1 (-24.5, 230) -> (-24.5, 242.5)
  line L2 (-24.5, 242.5) -> (-55, 242.5)
  line L3 (-55, 242.5) -> (-55, 230)
  line L4 (55, 230) -> (24.5, 230)
  line L5 (24.5, 230) -> (24.5, 242.5)
  line L6 (24.5, 242.5) -> (55, 242.5)
  line L7 (55, 242.5) -> (55, 230)
  line L8 (70, 194.5) -> (57.5, 194.5)
  line L9 (-55, -230) -> (-24.5, -230)
  line L10 (-24.5, -230) -> (-24.5, -242.5)
  line L11 (-24.5, -242.5) -> (-55, -242.5)
  line L12 (-55, -242.5) -> (-55, -230)
  line L13 (55, -230) -> (24.5, -230)
  line L14 (24.5, -230) -> (24.5, -242.5)
  line L15 (24.5, -242.5) -> (55, -242.5)
  line L16 (55, -242.5) -> (55, -230)
  circle A2 centre (17, 235) radius 2.25
  circle A3 centre (-17, 235) radius 2.25
  circle A4 centre (65, 184.5) radius 2.25
  circle A5 centre (17, -235) radius 2.25
  circle A6 centre (-17, -235) radius 2.25
  line L17 (-55, 242.5) -> (-55, 225) projected
  line L18 (57.5, 194.5) -> (57.5, 225)
  line L19 (57.5, 225) -> (70, 225)
  line L20 (70, 225) -> (70, 194.5)
  line L21 (33.7249, 144.5992) -> (33.7249, 139.1992) construction
  line L22 (33.7249, 141.8992) -> (65, 141.8992) construction
  point P0 (0, 0)
  point P1 (75, 58.3992)
  point P2 (75, 225)
  dimension "d117" = 4.5
  dimension "d119" = 4.5
  dimension "d120" = 30.5
  dimension "d122" = 10
  dimension "d125" = 7.5
  dimension "d126" = 7.5
  dimension "d127" = 7.5
  dimension "d128" = 7.5
  dimension "d133" = 12.5
  dimension "d170" = 5
  dimension "d190" = 10
  dimension "d191" = 10
  constraints: 44 end point, 8 equal length, 8 parallel, 7 centre point, 6 horizontal, 5 equal radius, 5 perpendicular, 3 vertical, 2 vertical alignment, 1 horizontal alignment, 1 midpoint, 1 point on line
  measures "d117" diameter of A0
  measures "d119" diameter of A1
  measures "d120" distance between parallel lines of L3 L1
  measures "d122" distance from line of L8 A4.centre
  measures "d125" distance from line of A2.centre L5
  measures "d126" distance from line of L1 A3.centre
  measures "d127" distance from line of A5.centre L14
  measures "d128" distance from line of L10 A6.centre
  measures "d133" distance of L0.end L1.end
  measures "d170" distance from line of L17.end L0
  measures "d190" horizontal distance of point (75, 58.399) A0.centre
  measures "d191" horizontal distance of point (75, 58.399) A0.centre
extrude "押し出し11" cut sketch "スケッチ11" against normal blind 3
sketch "スケッチ12" plane through (0, 0, 0) normal (0, 0, -1) x (-1, 0, 0)
  line L0 (-75, 225) -> (-55, 225) projected
  line L1 (-70, 194.5) -> (-75, 194.5)
  line L2 (-75, 194.5) -> (-75, 225)
  line L3 (-75, 225) -> (-70, 225)
  line L4 (-70, 225) -> (-70, 194.5)
  point P0 (0, 0)
  point P1 (-70, 225)
  constraints: 8 end point, 2 parallel, 1 horizontal, 1 perpendicular
extrude "押し出し12" cut sketch "スケッチ12" against normal blind 3
sketch "スケッチ13" plane through (0, 0, 0) normal (0, 0, -1) x (-1, 0, 0)
  line L0 (-42.22, -124.469) -> (-75, -124.469) projected
  line L1 (-75, -124.469) -> (-59, -124.469)
  line L2 (-59, -124.469) -> (-59, -114.469)
  line L3 (-59, -114.469) -> (-75, -114.469)
  line L4 (-75, -114.469) -> (-75, -124.469)
  point P0 (0, 0)
  point P1 (-35.0196, -115.1237)
  dimension "d139" = 16
  dimension "d140" = 10
  constraints: 8 end point, 2 parallel, 1 horizontal, 1 perpendicular, 1 other
  measures "d139" distance of L3.end L2.end
  measures "d140" distance of L2.end L1.end
extrude "押し出し13" add sketch "スケッチ13" against normal blind 3
sketch "スケッチ14" plane through (0, 0, 0) normal (0, 0, -1) x (-1, 0, 0)
  circle A0 centre (-65, -122.6) radius 2.25
  line L0 (-75, 58.3992) -> (-75, 194.5) projected
  line L1 (-59, -124.469) -> (-40.72, -124.469) projected
  line L2 (-75.0494, -117.1884) -> (-59.0494, -117.1884)
  line L3 (37.5, -137.6) -> (-61.5, -137.6) projected
  point P0 (0, 0)
  point P1 (-75, -225)
  point P2 (-42.22, -124.469)
  point P3 (-35.0196, -115.1237)
  point P4 (-75, 225)
  point P5 (-75, 194.5)
  point P6 (-75, 58.3992)
  point P7 (-75, -124.469)
  dimension "d143" = 4.5
  dimension "d144" = 10
  dimension "d209" = 15
  constraints: 2 end point, 1 centre point, 2 other
  measures "d143" diameter of A0
  measures "d209" distance from line of A0.centre L3
extrude "押し出し14" cut sketch "スケッチ14" against normal blind 3
sketch "スケッチ17" plane through (0, 0, 3) normal (0, 0, 1) x (1, 0, 0)
  line L0 (35.02, -101.4326) -> (34.74, -101.4326) projected
  line L1 (35.02, -91.9026) -> (35.02, -101.4326) projected
  line L2 (34.74, -91.9026) -> (35.02, -91.9026) projected
  line L3 (35.02, -81.0872) -> (34.74, -81.0872) projected
  line L4 (35.02, -71.5572) -> (35.02, -81.0872) projected
  line L5 (34.74, -71.5572) -> (35.02, -71.5572) projected
  line L6 (35.02, -60.7418) -> (34.74, -60.7418) projected
  line L7 (35.02, -51.2118) -> (35.02, -60.7418) projected
  line L8 (34.74, -51.2118) -> (35.02, -51.2118) projected
  line L9 (35.02, -40.3964) -> (34.74, -40.3964) projected
  line L10 (35.02, -30.8664) -> (35.02, -40.3964) projected
  line L11 (34.74, -30.8664) -> (35.02, -30.8664) projected
  line L12 (35.02, -20.051) -> (34.74, -20.051) projected
  line L13 (35.02, -10.521) -> (35.02, -20.051) projected
  line L14 (34.74, -10.521) -> (35.02, -10.521) projected
  line L15 (35.02, 0.2944) -> (34.74, 0.2944) projected
  line L16 (35.02, 9.8244) -> (35.02, 0.2944) projected
  line L17 (34.74, 9.8244) -> (35.02, 9.8244) projected
  line L18 (35.02, 20.6398) -> (34.74, 20.6398) projected
  line L19 (35.02, 30.1698) -> (35.02, 20.6398) projected
  line L20 (34.74, 30.1698) -> (35.02, 30.1698) projected
  line L21 (35.02, 40.9852) -> (34.74, 40.9852) projected
  line L22 (35.02, 50.5152) -> (35.02, 40.9852) projected
  line L23 (34.74, 50.5152) -> (35.02, 50.5152) projected
  line L24 (34.74, 40.9852) -> (34.74, 50.5152)
  line L25 (34.74, 20.6398) -> (35.02, 20.6398) projected
  line L26 (34.74, 30.1698) -> (34.74, 20.6398)
  line L27 (34.74, 9.8244) -> (34.74, 0.2944)
  line L28 (34.74, -10.521) -> (34.74, -20.051)
  line L29 (34.74, -30.8664) -> (34.74, -40.3964)
  line L30 (34.74, -51.2118) -> (34.74, -60.7418)
  line L31 (34.74, -71.5572) -> (34.74, -81.0872)
  line L32 (34.74, -91.9026) -> (34.74, -101.4326)
  point P0 (0, 0)
  point P1 (35.0196, -115.1237)
  point P2 (42.22, -101.4326)
  point P3 (40.72, -91.9026)
  point P4 (40.72, -81.0872)
  point P5 (40.72, -71.5572)
  point P6 (40.72, -60.7418)
  point P7 (40.72, -51.2118)
  point P8 (40.72, -40.3964)
  point P9 (40.72, -30.8664)
  point P10 (40.72, -20.051)
  point P11 (40.72, -10.521)
  point P12 (40.72, 0.2944)
  point P13 (39.12, 9.8244)
  point P14 (42.22, 20.6398)
  point P15 (42.22, 30.1698)
  point P16 (42.22, 40.9852)
  point P17 (42.22, 50.5152)
  point P18 (42.22, 9.8244)
  point P19 (42.22, -91.9026)
  point P20 (42.22, -81.0872)
  point P21 (42.22, -71.5572)
  point P22 (42.22, -60.7418)
  point P23 (42.22, -51.2118)
  point P24 (42.22, -40.3964)
  point P25 (42.22, -30.8664)
  point P26 (42.22, -20.051)
  point P27 (42.22, -10.521)
  point P28 (42.22, 0.2944)
  constraints: 16 end point, 6 perpendicular, 1 collinear, 1 vertical, 1 other
extrude "押し出し17" add sketch "スケッチ17" against normal up to surface (3 mm away) contours L3 L31 L5 L4 | L6 L30 L8 L7 | L9 L29 L11 L10 | L12 L28 L14 L13 | L15 L27 L17 L16 | L18 L26 L20 L19 | L21 L24 L23 L22
sketch "スケッチ18" plane through (0, 0, 3) normal (0, 0, 1) x (1, 0, 0)
  line L0 (-24.5, -242.5) -> (24.5, -242.5) construction
  line L1 (-24.5, -242.5) -> (24.5, -242.5) construction
  line L2 (0, -242.5) -> (0, -137.6) construction
  line L3 (61.5, -137.6) -> (-37.5, -137.6) construction
  line L4 (-78, -225) -> (-78, -132.6) construction
  line L5 (78, -225) -> (78, -132.6)
  line L6 (78, -132.6) -> (73, -132.6)
  line L7 (73, -132.6) -> (73, -225)
  line L8 (73, -225) -> (78, -225)
  point P0 (0, 0)
  point P1 (58.5, -140.6)
  point P2 (-36.2992, -140.6)
  point P3 (-55, -242.5)
  point P4 (55, -242.5)
  point P5 (-24.619, -122.5995)
  point P6 (42.22, -122.5995)
  point P7 (-22.419, -122.5995)
  point P8 (-37.5, -137.6)
  point P9 (-24.619, -140.6)
  dimension "d175" = 5
  constraints: 10 end point, 2 perpendicular, 2 symmetric about line, 1 horizontal, 1 midpoint, 1 vertical, 2 other
  measures "d175" distance of L5.end L6.end
extrude "押し出し18" add sketch "スケッチ18" against normal up to surface (3 mm away)
sketch "スケッチ20" plane through (0, 0, 3) normal (0, 0, 1) x (1, 0, 0)
  line L0 (42.22, 58.3992) -> (75, 58.3992) construction
  line L1 (42.22, 59.771) -> (42.22, 58.3992) construction
  line L2 (42.22, 59.771) -> (55, 59.771)
  line L3 (55, 59.771) -> (55, 58.3992)
  line L4 (55, 58.3992) -> (42.22, 58.3992)
  line L5 (42.22, 58.3992) -> (42.22, 59.771)
  line L6 (75, 58.3992) -> (75, 194.5) construction
  circle A0 centre (65, 68.3992) radius 2.25 construction
  point P0 (0, 0)
  dimension "d204" = 12.78
  dimension "d206" = 10
  constraints: 8 end point, 2 parallel, 1 horizontal, 1 perpendicular, 1 point on line
  measures "d204" distance of L1.start L2.end
  measures "d206" distance from line of L3 A0.centre
extrude "押し出し20" cut sketch "スケッチ20" against normal blind 10
equation "\"d7\" = d6"
equation "\"d8\" = d6"
equation "\"d9\" = d6"
equation "\"d12\" = d11"
equation "\"d32\" = d29"
equation "\"d48\" = d49"
equation "\"d52\" = d51"
equation "\"d53\" = d51"
equation "\"d54\" = d49"
equation "\"d56\" = d51"
equation "\"d57\" = d49"
equation "\"d58\" = d51"
equation "\"d59\" = d51"
equation "\"d84\" = d70 + d69"
